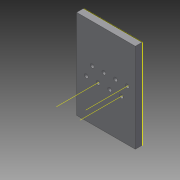
# Autodesk Inventor part: beep_rgb_ir
Saved by Autodesk Inventor 2014 (Build 180170000, 170)
## iProperties
Created: 2013-08-25
Part Number: beep_rgb_ir
Material: Generisch
Document SubType Name: Modeling
Designer: Felix
Density: 1 g/cm^3
Appearance: Vorgabe
Author: Felix
Autodesk Inventor part; units mm, degrees
ref_plane "YZ Plane" through (0, 0, 0) normal (1, 0, 0) x (0, 1, 0)
ref_plane "XZ Plane" through (0, 0, 0) normal (0, 1, 0) x (-1, 0, 0)
ref_plane "XY Plane" through (0, 0, 0) normal (0, 0, 1) x (1, 0, 0)
sketch "Skizze1" plane through (0, 0, 0) normal (0, 1, 0) x (-1, 0, 0)
  line L0 (0, 19.35) -> (0, 0)
  line L1 (12.735, 19.35) -> (0, 19.35)
  line L2 (12.735, 0) -> (12.735, 19.35)
  line L3 (0, 0) -> (12.735, 0)
  circle A0 centre (10.645, 8.43) radius 0.4064
  circle A1 centre (9.375, 10.97) radius 0.4064
  circle A2 centre (8.105, 8.43) radius 0.4064
  circle A3 centre (6.835, 10.97) radius 0.4064
  circle A4 centre (5.565, 8.43) radius 0.4064
  circle A5 centre (4.295, 10.97) radius 0.4064
  circle A6 centre (3.025, 8.43) radius 0.4064
  circle A7 centre (1.755, 10.97) radius 0.4064
  constraints: 8 centre point, 8 end point
extrude "Extrusion1" add sketch "Skizze1" along normal blind 1.5
sketch "Skizze5" plane through (0, 1.5, 0) normal (0, 1, 0) x (1, 0, 0)
  circle A0 centre (-1.755, -10.97) radius 0.4064 projected
  circle A1 centre (-3.025, -8.43) radius 0.4064 projected
  circle A2 centre (-4.295, -10.97) radius 0.4064 projected
  circle A3 centre (-5.565, -8.43) radius 0.4064 projected
  circle A4 centre (-6.835, -10.97) radius 0.4064 projected
  circle A5 centre (-8.105, -8.43) radius 0.4064 projected
  circle A6 centre (-9.375, -10.97) radius 0.4064 projected
  circle A7 centre (-10.645, -8.43) radius 0.4064 projected
  line L0 (0, -19.35) -> (0, 0) projected
  line L1 (0, 0) -> (-12.735, 0) projected
  line L2 (-12.735, 0) -> (-12.735, -19.35) projected
  line L3 (-12.735, -19.35) -> (0, -19.35) projected
  line L4 (0, 0) -> (-12.735, 0)
  line L5 (0, -19.35) -> (0, 0)
  line L6 (-12.735, 0) -> (-12.735, -19.35)
  line L7 (-12.735, -19.35) -> (0, -19.35)
  line L8 (-9.85, -15.125) -> (-9.85, -17.475)
  line L9 (-2.75, -15.125) -> (-9.85, -15.125)
  line L10 (-8.75, -1.42) -> (-8.75, -6.42)
  line L11 (-3.75, -1.42) -> (-8.75, -1.42)
  line L12 (-3.75, -6.42) -> (-3.75, -1.42)
  line L13 (-8.75, -6.42) -> (-3.75, -6.42)
  line L14 (-7.2, -17.4) -> (-7.2, -15.2)
  line L15 (-2.75, -17.475) -> (-2.75, -15.125)
  line L16 (-9.85, -17.475) -> (-2.75, -17.475)
  circle A8 centre (-9.375, -10.97) radius 0.4064
  circle A9 centre (-8.105, -8.43) radius 0.4064
  circle A10 centre (-6.835, -10.97) radius 0.4064
  circle A11 centre (-5.565, -8.43) radius 0.4064
  circle A12 centre (-1.755, -10.97) radius 0.4064
  circle A13 centre (-3.025, -8.43) radius 0.4064
  circle A14 centre (-4.295, -10.97) radius 0.4064
  circle A15 centre (-10.645, -8.43) radius 0.4064
  constraints: 26 end point, 8 centre point
